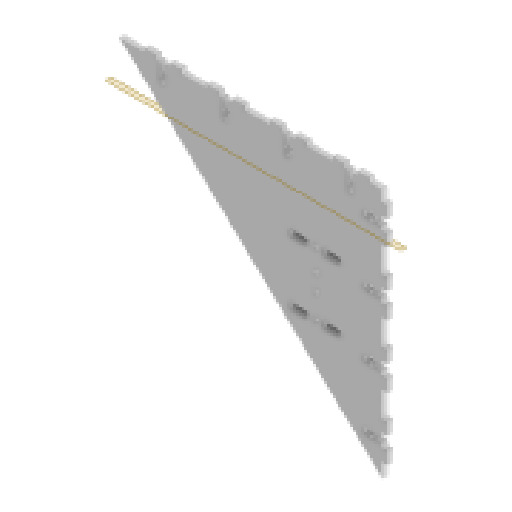
# Autodesk Inventor part: Ребро жёсткости для крепления хвоста
Saved by Autodesk Inventor 2023.2 (Build 272271030, 271C)
## iProperties
Created: 2024-03-15
Part Number: Ребро жёсткости для крепления хвоста
Material: Типовые
Document SubType Name: Modeling
Designer: I9232
Density: 1 g/cm^3
Appearance: По умолчанию
Author: I9232
Autodesk Inventor part; units mm, degrees
ref_plane "YZ Plane" through (0, 0, 0) normal (1, 0, 0) x (0, 1, 0)
ref_plane "XY Plane" through (0, 0, 0) normal (0, 0, 1) x (1, 0, 0)
sketch "Эскиз1" plane through (0, 0, 0) normal (0, 0, 1) x (1, 0, 0)
  line L0 (-190, 35) -> (20, 35)
  line L1 (20, 35) -> (20, -165)
  line L2 (20, -165) -> (-190, 35)
  dimension "d4" = 200
  dimension "d5" = 210
  constraints: 6 end point, 1 perpendicular
  measures "d4" distance of L0.end L1.end
  measures "d5" distance of L0.start L0.end
extrude "Выдавливание1" add sketch "Эскиз1" along normal mid plane 4
sketch "Эскиз2" plane through (-190, 35, 2) normal (0, 1, 0) x (1, 0, 0)
  line L0 (210, 0) -> (0, 0) projected
  line L1 (0, 4) -> (210, 4) projected
  line L2 (200, 0) -> (190, 0)
  line L3 (190, 0) -> (190, 4)
  line L4 (190, 4) -> (200, 4)
  line L5 (200, 4) -> (200, 0)
  line L6 (210, 4) -> (210, 0) projected
  line L7 (180, 0) -> (170, 0)
  line L8 (170, 0) -> (170, 4)
  line L9 (170, 4) -> (180, 4)
  line L10 (180, 4) -> (180, 0)
  line L11 (-300, 0) -> (-310, 0)
  line L12 (-310, 0) -> (-310, 4)
  line L13 (-310, 4) -> (-300, 4)
  line L14 (-300, 4) -> (-300, 0)
  line L15 (-320, 0) -> (-330, 0)
  line L16 (-330, 0) -> (-330, 4)
  line L17 (-330, 4) -> (-320, 4)
  line L18 (-320, 4) -> (-320, 0)
  line L19 (120, 0) -> (120, 4)
  line L20 (130, 0) -> (120, 0)
  line L21 (120, 4) -> (130, 4)
  line L22 (130, 4) -> (130, 0)
  line L23 (140, 0) -> (140, 4)
  line L24 (140, 4) -> (150, 4)
  line L25 (150, 4) -> (150, 0)
  line L26 (150, 0) -> (140, 0)
  line L27 (70, 0) -> (70, 4)
  line L28 (80, 0) -> (70, 0)
  line L29 (70, 4) -> (80, 4)
  line L30 (80, 4) -> (80, 0)
  line L31 (90, 0) -> (90, 4)
  line L32 (90, 4) -> (100, 4)
  line L33 (100, 4) -> (100, 0)
  line L34 (100, 0) -> (90, 0)
  line L35 (20, 0) -> (20, 4)
  line L36 (30, 0) -> (20, 0)
  line L37 (20, 4) -> (30, 4)
  line L38 (30, 4) -> (30, 0)
  line L39 (40, 0) -> (40, 4)
  line L40 (40, 4) -> (50, 4)
  line L41 (50, 4) -> (50, 0)
  line L42 (50, 0) -> (40, 0)
  point P0 (190, 2)
  point P1 (190, 2)
  point P2 (180, 2)
  point P3 (-310, 2)
  point P4 (-320, 2)
  point P5 (130, 2)
  point P6 (140, 2)
  point P7 (80, 2)
  point P8 (90, 2)
  point P9 (30, 2)
  point P10 (40, 2)
  point P11 (200, 4)
  point P12 (190, 0)
  point P13 (180, 4)
  point P14 (170, 0)
  point P15 (150, 0)
  point P16 (150, 4)
  point P17 (140, 4)
  point P18 (140, 0)
  point P19 (130, 0)
  point P20 (130, 4)
  point P21 (120, 0)
  point P22 (100, 0)
  point P23 (100, 4)
  point P24 (90, 4)
  point P25 (90, 0)
  point P26 (80, 0)
  point P27 (80, 4)
  point P28 (70, 0)
  point P29 (50, 0)
  point P30 (50, 4)
  point P31 (40, 4)
  point P32 (40, 0)
  point P33 (30, 0)
  point P34 (30, 4)
  point P35 (20, 0)
  dimension "d6" = 10
  dimension "d7" = 10
  dimension "d8" = 10
  dimension "d9" = 10
  dimension "d12" = 500
  dimension "d19" = 50
  constraints: 80 end point, 4 horizontal, 4 parallel, 4 point on line, 2 midpoint, 2 perpendicular, 72 other
  measures "d6" distance of L4.end L3.end
  measures "d7" distance between parallel lines of L5 L6
  measures "d8" distance of L9.end L8.end
  measures "d9" distance of point (190, 2) point (180, 2)
  measures "d12" distance of L2.start L11.start
  measures "d19" distance of L2.start L25.end
extrude "Выдавливание2" add sketch "Эскиз2" along normal blind 3 contours L0 L3 L1 L5 | L0 L8 L1 L10 | L0 L23 L1 L25 | L0 L19 L1 L22 | L0 L31 L1 L33 | L0 L27 L1 L30 | L0 L39 L1 L41 | L0 L35 L1 L38
sketch "Эскиз3" plane through (20, -165, 2) normal (1, 0, 0) x (0, 0, -1)
  line L0 (0, 0) -> (0, 200) projected
  line L1 (4, 0) -> (4, 200) projected
  line L2 (0, 11.5) -> (4, 11.5)
  line L3 (4, 11.5) -> (4, 21.5)
  line L4 (4, 21.5) -> (0, 21.5)
  line L5 (0, 21.5) -> (0, 11.5)
  line L6 (0, 0) -> (4, 0) projected
  line L7 (0, 31.5) -> (4, 31.5)
  line L8 (4, 31.5) -> (4, 41.5)
  line L9 (4, 41.5) -> (0, 41.5)
  line L10 (0, 41.5) -> (0, 31.5)
  line L11 (0, 61.5) -> (4, 61.5)
  line L12 (4, 61.5) -> (4, 71.5)
  line L13 (4, 71.5) -> (0, 71.5)
  line L14 (0, 71.5) -> (0, 61.5)
  line L15 (0, 81.5) -> (4, 81.5)
  line L16 (4, 81.5) -> (4, 91.5)
  line L17 (4, 91.5) -> (0, 91.5)
  line L18 (0, 91.5) -> (0, 81.5)
  line L19 (0, 111.5) -> (4, 111.5)
  line L20 (4, 111.5) -> (4, 121.5)
  line L21 (4, 121.5) -> (0, 121.5)
  line L22 (0, 121.5) -> (0, 111.5)
  line L23 (0, 131.5) -> (4, 131.5)
  line L24 (4, 131.5) -> (4, 141.5)
  line L25 (4, 141.5) -> (0, 141.5)
  line L26 (0, 141.5) -> (0, 131.5)
  line L27 (0, 161.5) -> (4, 161.5)
  line L28 (4, 161.5) -> (4, 171.5)
  line L29 (4, 171.5) -> (0, 171.5)
  line L30 (0, 171.5) -> (0, 161.5)
  line L31 (0, 181.5) -> (4, 181.5)
  line L32 (4, 181.5) -> (4, 191.5)
  line L33 (4, 191.5) -> (0, 191.5)
  line L34 (0, 191.5) -> (0, 181.5)
  point P0 (2, 165)
  point P1 (0, 41.5)
  point P2 (4, 31.5)
  point P3 (0, 21.5)
  point P4 (4, 11.5)
  point P5 (0, 191.5)
  point P6 (0, 171.5)
  point P7 (0, 141.5)
  point P8 (4, 121.5)
  point P9 (0, 121.5)
  point P10 (0, 111.5)
  point P11 (4, 111.5)
  point P12 (4, 91.5)
  point P13 (0, 91.5)
  point P14 (0, 71.5)
  dimension "d26" = 11.5
  dimension "d27" = 10
  dimension "d28" = 10
  dimension "d29" = 10
  dimension "d78" = 50
  constraints: 64 end point, 4 parallel, 4 point on line, 2 horizontal, 2 perpendicular, 1 vertical, 48 other
  measures "d26" distance between parallel lines of L2 L6
  measures "d27" distance of L3.end L2.end
  measures "d28" distance of L9.end L7.start
  measures "d29" distance between parallel lines of L7 L4
  measures "d78" distance of L2.start L11.start
extrude "Выдавливание3" add sketch "Эскиз3" along normal blind 4 contours L0 L4 L1 L2 | L0 L9 L1 L7 | L0 L13 L1 L11 | L0 L17 L1 L15 | L0 L21 L1 L19 | L0 L25 L1 L23 | L0 L29 L1 L27 | L0 L33 L1 L31
sketch "Эскиз4" plane through (0, 0, 2) normal (0, 0, 1) x (1, 0, 0)
  line L0 (5.1, -139.95) -> (5.1, -137.05)
  line L1 (20, -137.05) -> (20, -139.95)
  line L2 (20, -143.5) -> (20, -133.5) projected
  line L3 (5.1, -138.5) -> (20, -138.5) construction
  line L4 (20, -133.5) -> (20, -143.5) projected
  line L5 (10.1, -141.3) -> (11.9, -141.3)
  line L6 (11.9, -135.7) -> (10.1, -135.7)
  line L7 (20, -139.95) -> (11.9, -139.95)
  line L8 (10.1, -139.95) -> (5.1, -139.95)
  line L9 (10.1, -135.7) -> (10.1, -137.05)
  line L10 (10.1, -139.95) -> (10.1, -141.3)
  line L11 (11.9, -141.3) -> (11.9, -139.95)
  line L12 (11.9, -137.05) -> (11.9, -135.7)
  line L13 (5.1, -137.05) -> (10.1, -137.05)
  line L14 (11.9, -137.05) -> (20, -137.05)
  line L15 (-6.454, 35) -> (-3.546, 35)
  line L16 (-3.546, 20.1) -> (-6.446, 20.1)
  line L17 (-4.996, 20.1) -> (-5, 35) construction
  line L18 (0, 35) -> (-10, 35) projected
  line L19 (-2.196, 25.1) -> (-2.196, 26.9)
  line L20 (-7.796, 26.9) -> (-7.796, 25.1)
  line L21 (-6.446, 20.1) -> (-6.446, 25.1)
  line L22 (-6.454, 26.9) -> (-6.454, 35)
  line L23 (-7.796, 25.1) -> (-6.446, 25.1)
  line L24 (-3.546, 25.1) -> (-2.196, 25.1)
  line L25 (-2.196, 26.9) -> (-3.546, 26.9)
  line L26 (-6.454, 26.9) -> (-7.796, 26.9)
  line L27 (-3.546, 35) -> (-3.546, 26.9)
  line L28 (-3.546, 25.1) -> (-3.546, 20.1)
  line L29 (-53.546, 25.1) -> (-52.196, 25.1)
  line L30 (-57.796, 26.9) -> (-57.796, 25.1)
  line L31 (-56.454, 26.9) -> (-57.796, 26.9)
  line L32 (-52.196, 25.1) -> (-52.196, 26.9)
  line L33 (-52.196, 26.9) -> (-53.546, 26.9)
  line L34 (-54.996, 20.1) -> (-55, 35) construction
  line L35 (-53.546, 35) -> (-53.546, 26.9)
  line L36 (-56.454, 26.9) -> (-56.454, 35)
  line L37 (-56.454, 35) -> (-53.546, 35)
  line L38 (-53.546, 20.1) -> (-56.446, 20.1)
  line L39 (-53.546, 25.1) -> (-53.546, 20.1)
  line L40 (-56.446, 20.1) -> (-56.446, 25.1)
  line L41 (-57.796, 25.1) -> (-56.446, 25.1)
  line L42 (-103.546, 25.1) -> (-102.196, 25.1)
  line L43 (-107.796, 26.9) -> (-107.796, 25.1)
  line L44 (-106.454, 26.9) -> (-107.796, 26.9)
  line L45 (-102.196, 25.1) -> (-102.196, 26.9)
  line L46 (-102.196, 26.9) -> (-103.546, 26.9)
  line L47 (-104.996, 20.1) -> (-105, 35) construction
  line L48 (-103.546, 35) -> (-103.546, 26.9)
  line L49 (-106.454, 26.9) -> (-106.454, 35)
  line L50 (-106.454, 35) -> (-103.546, 35)
  line L51 (-103.546, 20.1) -> (-106.446, 20.1)
  line L52 (-103.546, 25.1) -> (-103.546, 20.1)
  line L53 (-106.446, 20.1) -> (-106.446, 25.1)
  line L54 (-107.796, 25.1) -> (-106.446, 25.1)
  line L55 (-153.546, 25.1) -> (-152.196, 25.1)
  line L56 (-157.796, 26.9) -> (-157.796, 25.1)
  line L57 (-156.454, 26.9) -> (-157.796, 26.9)
  line L58 (-152.196, 25.1) -> (-152.196, 26.9)
  line L59 (-152.196, 26.9) -> (-153.546, 26.9)
  line L60 (-154.996, 20.1) -> (-155, 35) construction
  line L61 (-153.546, 35) -> (-153.546, 26.9)
  line L62 (-156.454, 26.9) -> (-156.454, 35)
  line L63 (-156.454, 35) -> (-153.546, 35)
  line L64 (-153.546, 20.1) -> (-156.446, 20.1)
  line L65 (-153.546, 25.1) -> (-153.546, 20.1)
  line L66 (-156.446, 20.1) -> (-156.446, 25.1)
  line L67 (-157.796, 25.1) -> (-156.446, 25.1)
  line L68 (10.1, -91.3) -> (11.9, -91.3)
  line L69 (11.9, -91.3) -> (11.9, -89.95)
  line L70 (10.1, -89.95) -> (10.1, -91.3)
  line L71 (5.1, -88.5) -> (20, -88.5) construction
  line L72 (11.9, -87.05) -> (20, -87.05)
  line L73 (20, -87.05) -> (20, -89.95)
  line L74 (20, -89.95) -> (11.9, -89.95)
  line L75 (10.1, -85.7) -> (10.1, -87.05)
  line L76 (11.9, -85.7) -> (10.1, -85.7)
  line L77 (5.1, -87.05) -> (10.1, -87.05)
  line L78 (5.1, -89.95) -> (5.1, -87.05)
  line L79 (10.1, -89.95) -> (5.1, -89.95)
  line L80 (11.9, -87.05) -> (11.9, -85.7)
  line L81 (10.1, -41.3) -> (11.9, -41.3)
  line L82 (11.9, -41.3) -> (11.9, -39.95)
  line L83 (10.1, -39.95) -> (10.1, -41.3)
  line L84 (5.1, -38.5) -> (20, -38.5) construction
  line L85 (11.9, -37.05) -> (20, -37.05)
  line L86 (20, -37.05) -> (20, -39.95)
  line L87 (20, -39.95) -> (11.9, -39.95)
  line L88 (10.1, -35.7) -> (10.1, -37.05)
  line L89 (11.9, -35.7) -> (10.1, -35.7)
  line L90 (5.1, -37.05) -> (10.1, -37.05)
  line L91 (5.1, -39.95) -> (5.1, -37.05)
  line L92 (10.1, -39.95) -> (5.1, -39.95)
  line L93 (11.9, -37.05) -> (11.9, -35.7)
  line L94 (10.1, 8.7) -> (11.9, 8.7)
  line L95 (11.9, 8.7) -> (11.9, 10.05)
  line L96 (10.1, 10.05) -> (10.1, 8.7)
  line L97 (5.1, 11.5) -> (20, 11.5) construction
  line L98 (11.9, 12.95) -> (20, 12.95)
  line L99 (20, 12.95) -> (20, 10.05)
  line L100 (20, 10.05) -> (11.9, 10.05)
  line L101 (10.1, 14.3) -> (10.1, 12.95)
  line L102 (11.9, 14.3) -> (10.1, 14.3)
  line L103 (5.1, 12.95) -> (10.1, 12.95)
  line L104 (5.1, 10.05) -> (5.1, 12.95)
  line L105 (10.1, 10.05) -> (5.1, 10.05)
  line L106 (11.9, 12.95) -> (11.9, 14.3)
  point P0 (0, 0)
  point P1 (11.9, -136.375)
  point P2 (11.9, -140.625)
  point P3 (-7.125, 26.9)
  point P4 (-57.125, 26.9)
  point P5 (-107.125, 26.9)
  point P6 (-157.125, 26.9)
  point P7 (11.9, -90.625)
  point P8 (20, -83.5)
  point P9 (20, -93.5)
  point P10 (11.9, -86.375)
  point P11 (11.9, -40.625)
  point P12 (20, -33.5)
  point P13 (20, -43.5)
  point P14 (11.9, -36.375)
  point P15 (11.9, 9.375)
  point P16 (20, 16.5)
  point P17 (20, 6.5)
  point P18 (11.9, 13.625)
  dimension "d39" = 2.9
  dimension "d40" = 5.6
  dimension "d41" = 1.8
  dimension "d43" = 5
  dimension "d44" = 8.1
  dimension "d45" = 8.1
  dimension "d46" = 1.35
  dimension "d54" = 2.9
  dimension "d55" = 1.8
  dimension "d56" = 5.6
  dimension "d57" = 1.35
  dimension "d58" = 5
  dimension "d59" = 8.1
  dimension "d62" = 50
  dimension "d71" = 50
  constraints: 208 end point, 24 parallel, 9 midpoint, 9 perpendicular, 7 horizontal, 1 vertical, 177 other
  measures "d39" distance of L0.start L0.end
  measures "d40" distance between parallel lines of L6 L5
  measures "d41" distance of L6.start L6.end
  measures "d43" distance of L9.end L0.end
  measures "d44" distance from line of L1 point (11.9, -136.375)
  measures "d45" distance from line of L2 point (11.9, -140.625)
  measures "d46" distance of L8.start L5.start
  measures "d54" distance of L16.start L16.end
  measures "d55" distance of L20.start L20.end
  measures "d56" distance of L19.end L20.start
  measures "d57" distance of L20.end L21.end
  measures "d58" distance of L16.end L21.end
  measures "d59" distance from line of L18 point (-7.125, 26.9)
  measures "d62" distance of L19.start L29.end
  measures "d71" distance of L7.end L69.end
extrude "Выдавливание4" cut sketch "Эскиз4" against normal up to surface (4 mm away)
sketch "Эскиз5" plane through (0, 0, -2) normal (0, 0, -1) x (-1, 0, 0)
  line L0 (39.5115, -83.4868) -> (39.5115, -79.4868)
  line L1 (39.5115, -79.4868) -> (52.8449, -79.4868)
  line L2 (52.8449, -79.4868) -> (52.8449, -83.4868)
  line L3 (52.8449, -83.4868) -> (39.5115, -83.4868)
  line L4 (12.8449, -79.4868) -> (26.1782, -79.4868)
  line L5 (26.1782, -79.4868) -> (26.1782, -83.4868)
  line L6 (26.1782, -83.4868) -> (12.8449, -83.4868)
  line L7 (12.8449, -83.4868) -> (12.8449, -79.4868)
  line L8 (26.1782, -29.2868) -> (26.1782, -33.2868)
  line L9 (26.1782, -33.2868) -> (12.8449, -33.2868)
  line L10 (12.8449, -33.2868) -> (12.8449, -29.2868)
  line L11 (12.8449, -29.2868) -> (26.1782, -29.2868)
  line L12 (52.8449, -33.2868) -> (39.5115, -33.2868)
  line L13 (39.5115, -33.2868) -> (39.5115, -29.2868)
  line L14 (39.5115, -29.2868) -> (52.8449, -29.2868)
  line L15 (52.8449, -29.2868) -> (52.8449, -33.2868)
  line L16 (56.3449, -88.8868) -> (56.3449, -23.8868)
  line L17 (56.3449, -23.8868) -> (9.3449, -23.8868)
  line L18 (9.3449, -23.8868) -> (9.3449, -88.8868)
  line L19 (9.3449, -88.8868) -> (56.3449, -88.8868)
  circle A0 centre (32.8449, -62.8868) radius 1
  circle A1 centre (32.8449, -48.8868) radius 1
  circle A2 centre (32.8449, -81.4868) radius 1.5
  circle A3 centre (32.8449, -31.2868) radius 1.5
  point P0 (0, 0)
  constraints: 40 end point, 4 centre point
extrude "Выдавливание5" cut sketch "Эскиз5" against normal up to surface (4 mm away) contours L0 L1 L2 L3 | L4 L5 L6 L7 | L8 L9 L10 L11 | L12 L13 L14 L15 | A0 | A1 | A2 | A3
